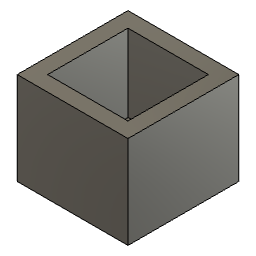
FOOT_CAP (Autodesk Fusion 360 design; units mm, degrees)
Autodesk Fusion 360 part; units mm, degrees
sketch "Sketch1" plane through (0, 0, 0) normal (0, 1, 0) x (1, 0, 0)
  line L0 (18.2, 18.2) -> (-18.2, 18.2)
  line L1 (-18.2, 18.2) -> (-18.2, -18.2)
  line L2 (-18.2, -18.2) -> (18.2, -18.2)
  line L3 (18.2, -18.2) -> (18.2, 18.2)
  line L4 (18.2, 18.2) -> (-18.2, -18.2) construction
  line L5 (-18.2, 18.2) -> (18.2, -18.2) construction
  line L6 (-18.2, 18.2) -> (18.2, 18.2)
  line L7 (18.2, 18.2) -> (18.2, 13.2)
  line L8 (18.2, 13.2) -> (-18.2, 13.2)
  line L9 (-18.2, 13.2) -> (-18.2, 18.2)
  line L10 (18.2, -18.2) -> (-18.2, -18.2)
  line L11 (-18.2, -18.2) -> (-18.2, -13.2)
  line L12 (-18.2, -13.2) -> (18.2, -13.2)
  line L13 (18.2, -13.2) -> (18.2, -18.2)
  line L14 (-18.2, 13.2) -> (-13.2, 13.2)
  line L15 (-13.2, 13.2) -> (-13.2, -13.2)
  line L16 (-13.2, -13.2) -> (-18.2, -13.2)
  line L17 (-18.2, -13.2) -> (-18.2, 13.2)
  line L18 (18.2, 13.2) -> (13.2, 13.2)
  line L19 (13.2, 13.2) -> (13.2, -13.2)
  line L20 (13.2, -13.2) -> (18.2, -13.2)
  line L21 (18.2, -13.2) -> (18.2, 13.2)
  dimension "d4" = 36.4
  dimension "d5" = 36.4
  dimension "d6" = 5
  dimension "d7" = 5
  dimension "d8" = 5
  dimension "d9" = 5
  constraint horizontal L0
  constraint perpendicular L0 L1
  constraint parallel L0 L2
  constraint parallel L1 L3
  constraint coincident L4 origin
  constraint coincident L5 origin
  constraint horizontal L6
  constraint vertical L7
  constraint horizontal L8
  constraint vertical L9
  constraint horizontal L10
  constraint vertical L11
  constraint horizontal L12
  constraint vertical L13
  constraint horizontal L14
  constraint vertical L15
  constraint horizontal L16
  constraint vertical L17
  constraint horizontal L18
  constraint vertical L19
  constraint horizontal L20
  constraint vertical L21
  measures "d4" distance of L1.end L2.end
  measures "d5" distance of L0.end L1.end
  measures "d6" distance of L0.end L8.end
  measures "d7" distance of L2.end L12.end
  measures "d8" distance of L8.end L14.end
  measures "d9" distance of L7.end L18.end
extrude "Extrude1" add sketch "Sketch1" along normal blind 25.4 contours L0 L1 L3 L6 L7 L8 L9 L14 L18 | L3 L8 L12 L18 L19 L20 L21 | L1 L8 L12 L14 L15 L16 L17 | L1 L2 L3 L10 L11 L12 L13 L16 L20
extrude "Extrude2" add 1 faces at (4.4, 0, 16.5333) along direction (0, -1, 0) blind 5
extrude "Extrude3" add sketch "Sketch1" against normal blind 5 contours L8 L12 L15 L19
equation "ONEINCH = 25.4 mm"
equation "TOLERANCE = 0.5 mm"
equation "WALL_THICKNESS = 5 mm"
equation "d4 = ONEINCH + ( 2 * TOLERANCE ) + ( WALL_THICKNESS * 2 )"
equation "d5 = ONEINCH + ( 2 * TOLERANCE ) + ( WALL_THICKNESS * 2 )"
equation "d6 = WALL_THICKNESS"
equation "d7 = WALL_THICKNESS"
equation "d8 = WALL_THICKNESS"
equation "d9 = WALL_THICKNESS"
equation "d10 = ONEINCH"
equation "d12 = WALL_THICKNESS"
